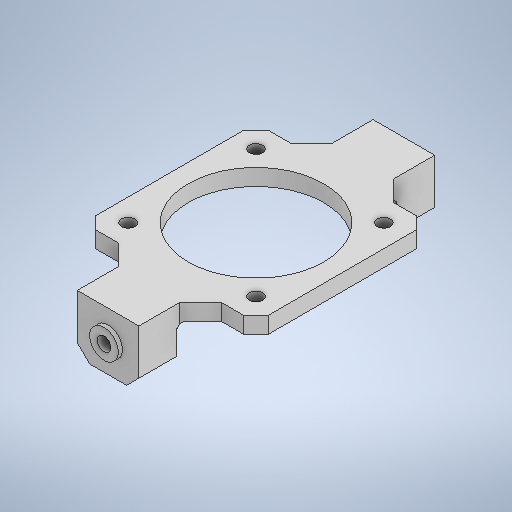
# Autodesk Inventor part: PingPongLauncherWinkel
Saved by Autodesk Inventor 2025 (Build 290162010, 162A)
## iProperties
Created: 2024-10-07
Part Number: PingPongLauncherWinkel
Material: Generisch
Document SubType Name: Modeling
Designer: max-h
Density: 1 g/cm^3
Appearance: Vorgabe
Author: max-h
Autodesk Inventor part; units mm, degrees
ref_plane "YZ Plane" through (0, 0, 0) normal (1, 0, 0) x (0, 1, 0)
ref_plane "XZ Plane" through (0, 0, 0) normal (0, 1, 0) x (-1, 0, 0)
ref_plane "XY Plane" through (0, 0, 0) normal (0, 0, 1) x (1, 0, 0)
sketch "Skizze24" plane through (0, 0, 0) normal (0, 1, 0) x (-1, 0, 0)
  line L0 (21, 21) -> (7.5, 21)
  line L1 (-21, 21) -> (-21, -21)
  line L2 (-21, -21) -> (-7.5, -21)
  line L3 (21, -21) -> (21, 21)
  circle A0 centre (0, 0) radius 16.5
  line L4 (29.4, 0) -> (-29.4, 0) projected
  line L5 (0, -50.4) -> (0, 50.4) projected
  circle A1 centre (15.555, 15.555) radius 1.625
  circle A2 centre (15.555, -15.555) radius 1.625
  circle A3 centre (-15.555, -15.555) radius 1.625
  circle A4 centre (-15.555, 15.555) radius 1.625
  line L6 (15.555, 15.555) -> (-15.555, 15.555) construction
  line L7 (-15.555, 15.555) -> (-15.555, -15.555) construction
  line L8 (-15.555, -15.555) -> (15.555, -15.555) construction
  line L9 (15.555, -15.555) -> (15.555, 15.555) construction
  line L10 (7.5, 36) -> (-7.5, 36)
  line L11 (-7.5, 36) -> (-7.5, 21)
  line L12 (7.5, 21) -> (7.5, 36)
  line L13 (-7.5, -21) -> (-7.5, -36)
  line L14 (-7.5, -36) -> (7.5, -36)
  line L15 (7.5, -36) -> (7.5, -21)
  line L16 (-7.5, 21) -> (-21, 21)
  line L17 (7.5, -21) -> (21, -21)
  dimension "d120" = 42
  dimension "d121" = 33
  dimension "d122" = 3.25
  dimension "d123" = 31.11
  dimension "d126" = 15
  dimension "d127" = 15
  dimension "d128" = 13.5
  constraints: 32 end point, 9 parallel, 5 centre point, 5 coincident, 5 perpendicular, 4 equal length, 4 horizontal, 3 equal radius, 1 point on line, 6 other
  measures "d120" distance of L3.start L0.start
  measures "d121" diameter of A0
  measures "d122" diameter of A1
  measures "d123" distance of L8.end L6.start
  measures "d126" distance of L0.end L10.start
  measures "d127" distance of L10.start L10.end
  measures "d128" distance of L0.start L0.end
extrude "Extrusion24" add sketch "Skizze24" along normal blind 4 contours L3 L4 A0 L5 L10 L12 L0 | L3 L17 L15 L14 L5 A0 L4 | L5 A0 L4 L1 L16 L11 L10 | L5 L14 L13 L2 L1 L4 A0
sketch "Skizze25" plane through (0, 0, 0) normal (0, -1, 0) x (1, 0, 0)
  line L0 (7.5, 36) -> (7.5, 21) projected
  line L1 (-7.5, 21) -> (-7.5, 36) projected
  line L2 (7.5, 36) -> (-7.5, 36)
  line L3 (-7.5, 36) -> (-7.5, 26.75)
  line L4 (-7.5, 26.75) -> (7.5, 26.75)
  line L5 (7.5, 26.75) -> (7.5, 36)
  line L6 (7.5, -36) -> (-7.5, -36)
  line L7 (-7.5, -36) -> (-7.5, -26.75)
  line L8 (-7.5, -26.75) -> (7.5, -26.75)
  line L9 (7.5, -26.75) -> (7.5, -36)
  point P0 (0, 0)
  point P1 (-7.5, 36)
  point P2 (7.5, 26.75)
  dimension "d129" = 9.25
  dimension "d130" = 9.25
  constraints: 16 end point, 4 parallel, 3 point on line, 2 horizontal, 2 perpendicular
  measures "d129" distance between parallel lines of L6 L8
  measures "d130" distance between parallel lines of L2 L4
extrude "Extrusion25" add sketch "Skizze25" along normal blind 10
sketch "Skizze26" plane through (-7.5, 4, 36) normal (0, 0, 1) x (1, 0, 0)
  circle A0 centre (7.5, -7) radius 1.675
  line L0 (-9, 0) -> (24, 0) projected
  line L1 (7.5, 0) -> (7.5, -13.9101)
  line L2 (0, -14) -> (0, 0) projected
  line L3 (0, -7) -> (15.6151, -7)
  point P0 (7.5, -4)
  dimension "d133" = 3.35
  constraints: 4 end point, 2 midpoint, 2 point on line, 1 centre point, 1 horizontal, 1 vertical
  measures "d133" diameter of A0
extrude "Extrusion26" cut sketch "Skizze26" against normal through all contours L3 L1 A0 | A0 L1 L3 | L1 L3 A0 | A0 L3 L1
chamfer "Fasen5" distance 3 angle 45 8 edges at (21, 2, -21) (21, 2, 21) (-21, 2, 21) (-21, 2, -21) (7.5, -10, -31.375) (-7.5, -10, -31.375) (-7.5, -10, 31.375) (7.5, -10, 31.375)
chamfer "Fasen6" distance 1.25 angle 45 2 edges at (0, 0, -26.75) (0, 0, 26.75)
chamfer "Fasen7" distance 5 angle 45 4 edges at (7.5, 2, -21) (7.5, 2, 21) (-7.5, 2, 21) (-7.5, 2, -21)
sketch "Skizze29" plane through (7.5, 4, -36) normal (0, 0, -1) x (-1, 0, 0)
  circle A0 centre (7.5, -7) radius 1.675 projected
  circle A1 centre (7.5, -7) radius 1.675
  circle A2 centre (7.5, -7) radius 3.5
  point P0 (7.5, -4)
  dimension "d151" = 7
  constraints: 2 centre point, 2 coincident, 1 concentric
  measures "d151" diameter of A2
extrude "Extrusion29" add sketch "Skizze29" along normal blind 1
sketch "Skizze30" plane through (-7.5, 4, 36) normal (0, 0, 1) x (1, 0, 0)
  circle A0 centre (7.5, -7) radius 1.675 projected
  circle A1 centre (7.5, -7) radius 3.5
  point P0 (7.5, -4)
  dimension "d154" = 7
  constraints: 1 centre point, 1 coincident
  measures "d154" diameter of A1
extrude "Extrusion30" add sketch "Skizze30" along normal blind 1
